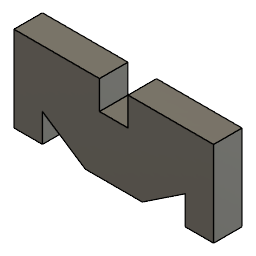
Exercise _6_Problem (Autodesk Fusion 360 design; units mm, degrees)
part number: 2026-05-20-10-44-42-134
Autodesk Fusion 360 part; units mm, degrees
sketch "Sketch1" plane through (0, 0, 0) normal (0, 1, 0) x (1, 0, 0)
  line L0 (35, -5) -> (-35, -5)
  line L1 (-35, -5) -> (-35, 5)
  line L2 (-35, 5) -> (35, 5)
  line L3 (35, 5) -> (35, -5)
  line L4 (35, -5) -> (-35, 5) construction
  line L5 (-35, -5) -> (35, 5) construction
  dimension "d1" = 70
  dimension "d2" = 10
  constraint horizontal L0
  constraint perpendicular L0 L1
  constraint parallel L0 L2
  constraint parallel L1 L3
  constraint coincident L4 origin
  constraint coincident L5 origin
  measures "d1" distance of L1.end L2.end
  measures "d2" distance of L0.end L1.end
extrude "Extrude1" add sketch "Sketch1" along normal blind 30
sketch "Sketch2" plane through (0, 0, 5) normal (0, 0, 1) x (1, 0, 0)
  line L0 (-35, 0) -> (35, 0)
  line L1 (35, 0) -> (35, 30)
  line L2 (35, 30) -> (-35, 30)
  line L3 (-35, 30) -> (-35, 0)
  line L4 (0, 30) -> (-5, 30)
  line L5 (0, 30) -> (5, 30)
  line L6 (-25, 0) -> (-25, 10)
  line L7 (-25, 10) -> (-10, 0)
  line L8 (25, 0) -> (25, 10)
  line L9 (25, 10) -> (10, 0)
  line L10 (-25, 0) -> (-10, 0)
  line L11 (10, 0) -> (25, 0)
  line L12 (-5, 30) -> (-5, 20)
  line L13 (-5, 20) -> (5, 20)
  line L14 (5, 20) -> (5, 30)
  line L15 (-35, 30) -> (-35, 0)
  line L16 (-25, 0) -> (-35, 0)
  line L17 (-35, 30) -> (35, 30)
  line L18 (35, 30) -> (35, 0)
  line L19 (35, 0) -> (-10, 0)
  dimension "d5" = 5
  dimension "d6" = 5
  dimension "d7" = 10
  dimension "d8" = 10
  dimension "d9" = 10
  dimension "d10" = 15
  dimension "d13" = 10
  constraint parallel L2 L4
  constraint parallel L2 L5
  constraint perpendicular L0 L8
  constraint coincident L0 L9.end
  constraint perpendicular L6 L10
  constraint perpendicular L6 L11
  constraint perpendicular L4 L12
  constraint perpendicular L12 L13
  constraint perpendicular L2 L14
  constraint coincident L2.end L3.start
  constraint coincident L0.start L3.end
  constraint perpendicular L3 L16
  constraint coincident L1.end L2.start
  constraint coincident L0.end L1.start
  constraint perpendicular L18 L19
  measures "d5" distance of L4.start L4.end
  measures "d6" distance of L4.start L5.end
  measures "d7" distance of L0.end L8.start
  measures "d8" distance of L0.start L6.start
  measures "d9" distance of L6.start L6.end
  measures "d10" distance of L6.start L7.end
  measures "d13" distance of L8.start L8.end
extrude "Extrude2" cut sketch "Sketch2" against normal blind 10 contours L0 L6 L7 L10 | L2 L4 L5 L12 L13 L14 L17 | L0 L8 L9 L11 L19
